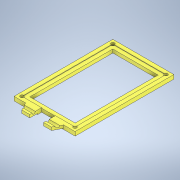
# Autodesk Inventor part: 筛网
Saved by Autodesk Inventor 2022 (Build 260153000, 153)
## iProperties
Created: 2022-05-21
Part Number: 筛网
Material: 常规
Document SubType Name: Modeling
Designer: zhcne
Density: 1 g/cm^3
Appearance: 默认
Author: zhcne
Autodesk Inventor part; units mm, degrees
ref_plane "YZ Plane" through (0, 0, 0) normal (1, 0, 0) x (0, 1, 0)
ref_plane "XZ Plane" through (0, 0, 0) normal (0, 1, 0) x (-1, 0, 0)
ref_plane "XY Plane" through (0, 0, 0) normal (0, 0, 1) x (1, 0, 0)
sketch "草图1" plane through (0, 0, 0) normal (0, 1, 0) x (-1, 0, 0)
  line L0 (30.9, 50) -> (30.9, -50)
  line L1 (30.9, -50) -> (-30.9, -50)
  line L2 (-30.9, -50) -> (-30.9, 50)
  line L3 (-30.9, 50) -> (30.9, 50)
  line L4 (0, 0) -> (5.4307, 0)
  line L5 (0, 0) -> (0, 9.1176)
  line L6 (22.9, 42) -> (-22.9, 42)
  line L7 (-22.9, 42) -> (-22.9, -42)
  line L8 (-22.9, -42) -> (22.9, -42)
  line L9 (22.9, -42) -> (22.9, 42)
  circle A0 centre (26.9, 46) radius 1.75
  circle A1 centre (26.9, -46) radius 1.75
  circle A2 centre (-26.9, 46) radius 1.75
  circle A3 centre (-26.9, -46) radius 1.75
  dimension "d0" = 100
  dimension "d1" = 61.8
  dimension "d2" = 8
  dimension "d3" = 8
  dimension "d4" = 3.5
  dimension "d5" = 4
  dimension "d6" = 4
  dimension "d9" = 92
  dimension "d12" = 53.8
  constraints: 20 end point, 4 centre point, 4 perpendicular, 3 horizontal, 3 vertical, 2 parallel, 10 other
  measures "d0" distance of L0.start L0.end
  measures "d1" distance of L0.end L1.end
  measures "d2" distance between parallel lines of L1 L8
  measures "d3" distance between parallel lines of L0 L9
  measures "d4" diameter of A0
  measures "d5" distance from line of L0 A0.centre
  measures "d6" distance from line of L3 A0.centre
  measures "d9" distance of A0.centre A1.centre
  measures "d12" distance of A0.centre A2.centre
extrude "拉伸1" add sketch "草图1" along normal blind 4
sketch "草图2" plane through (0, 4, 0) normal (0, 1, 0) x (1, 0, 0)
  line L0 (-30.9, -50) -> (30.9, -50) construction
  line L1 (-19.2161, -50) -> (-15, -58)
  line L2 (-15, -58) -> (15, -58)
  line L3 (15, -58) -> (19.2161, -50)
  line L4 (0, 0) -> (0, -17.0054)
  line L5 (-19.2161, -50) -> (19.2161, -50)
  dimension "d17" = 8
  dimension "d18" = 30
  constraints: 10 end point, 2 point on line, 1 horizontal, 1 parallel, 1 vertical, 1 other
  measures "d17" distance between parallel lines of L0 L2
  measures "d18" distance of L1.end L2.end
extrude "拉伸2" add sketch "草图2" against normal blind 3
sketch "草图3" plane through (0, 0, 0) normal (1, 0, 0) x (0, 1, 0)
  line L0 (4, 50) -> (4, 58) construction
  circle A0 centre (4, 54) radius 1.6
  point P0 (0, 0)
  dimension "d21" = 3.2
  constraints: 1 centre point, 1 midpoint
  measures "d21" diameter of A0
extrude "拉伸3" cut sketch "草图3" along normal mid plane 40
sketch "草图4" plane through (0, 4, 0) normal (0, 1, 0) x (1, 0, 0)
  line L0 (15, -58) -> (-15, -58) construction
  line L1 (-7, -58) -> (-7, -46)
  line L2 (-7, -46) -> (7, -46)
  line L3 (-30.9, -50) -> (30.9, -50) projected
  line L4 (7, -46) -> (7, -58)
  line L5 (7, -58) -> (-7, -58)
  line L6 (0, 0) -> (0, -70.1982)
  dimension "d26" = 12
  dimension "d27" = 14
  constraints: 10 end point, 3 perpendicular, 1 parallel, 1 point on line, 1 vertical, 1 other
  measures "d26" distance of L1.start L1.end
  measures "d27" distance of L1.end L2.end
extrude "拉伸4" cut sketch "草图4" against normal blind 40
sketch "草图5" plane through (0, 4, 0) normal (0, 1, 0) x (1, 0, 0)
  circle A0 centre (-26.9, -46) radius 1.75 projected
  circle A1 centre (26.9, 46) radius 1.75 projected
  line L0 (-26.9, -46) -> (26.9, -46)
  line L1 (26.9, -46) -> (26.9, 46)
  line L2 (26.9, 46) -> (-26.9, 46)
  line L3 (-26.9, 46) -> (-26.9, -46)
  point P0 (0, 0)
  constraints: 8 end point, 2 parallel, 1 horizontal, 1 perpendicular
extrude "拉伸5" cut sketch "草图5" against normal blind 0.5 contours L0 L3 A0 | A0 L3 L2 A1 L1 L0 | A1 L2 L1 picked at (-26.2832, -45.0184) picked at (25.748, 45.8702)
